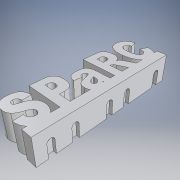
# Autodesk Inventor part: RGB Stand
Saved by Autodesk Inventor 2016 (Build 200138000, 138)
## iProperties
Created: 2015-11-06
Part Number: RGB Stand
Material: PPS Plastic
Document SubType Name: Modeling
Designer: Matthew
Density: 1.637 g/cm^3
Appearance: Smooth - White
Author: Matthew
## iProperties of the stored document RGB Stand_3DPrint.ipt
Created: 2015-11-06
Part Number: RGB Stand_3DPrint
Material: Generic
Document SubType Name: Modeling
Designer: Matthew
Density: 1 g/cm^3
Appearance: Default
Author: Matthew
Autodesk Inventor part; units mm, degrees
ref_plane "YZ Plane" through (0, 0, 0) normal (1, 0, 0) x (0, 1, 0)
ref_plane "XZ Plane" through (0, 0, 0) normal (0, 1, 0) x (-1, 0, 0)
ref_plane "XY Plane" through (0, 0, 0) normal (0, 0, 1) x (1, 0, 0)
sketch "Sketch1" plane through (0, 0, 0) normal (0, 1, 0) x (-1, 0, 0)
  line L0 (0, 0) -> (0, -279.4)
  line L1 (-0.0603, 0.0541) -> (-0.0603, -814.8468) construction
  line L2 (-0.0603, -814.8468) -> (-6674.4868, -814.8468) construction
  line L3 (-6674.4868, -814.8468) -> (-6674.4868, 0.0541) construction
  line L4 (-6674.4868, 0.0541) -> (-0.0603, 0.0541) construction
  line L5 (-49.463, -2.5788) -> (-48.1465, -18.4459)
  spline S0 degree 2 poles (-48.1465, -18.4459) (-53.3432, -18.9309) (-56.0454, -20.5246) knots 0 0 0 1 1 1
  spline S1 degree 2 poles (-56.0454, -20.5246) (-60.4106, -23.1575) (-60.4106, -27.9384) knots 0 0 0 1 1 1
  spline S2 degree 2 poles (-60.4106, -27.9384) (-60.4106, -31.4721) (-55.9068, -35.3523) (-52.9967, -35.3523) knots 0 0 0 1 2 2 2
  spline S3 degree 2 poles (-52.9967, -35.3523) (-50.2252, -35.3523) (-48.0079, -33.4815) knots 0 0 0 1 1 1
  spline S4 degree 2 poles (-48.0079, -33.4815) (-45.7907, -31.68) (-43.7813, -24.959) knots 0 0 0 1 1 1
  spline S5 degree 2 poles (-43.7813, -24.959) (-40.5248, -14.0114) (-35.051, -9.2998) knots 0 0 0 1 1 1
  spline S6 degree 2 poles (-35.051, -9.2998) (-29.5772, -4.5882) (-21.124, -4.5882) knots 0 0 0 1 1 1
  spline S7 degree 2 poles (-21.124, -4.5882) (-15.5809, -4.5882) (-5.742, -9.4384) (-0.0603, -19.1388) (-0.0603, -27.592) knots 0 0 0 1 2 3 3 3
  spline S8 degree 2 poles (-0.0603, -27.592) (-0.0603, -37.916) (-10.315, -48.7942) (-21.5398, -49.8336) knots 0 0 0 1 2 2 2
  line L6 (-21.5398, -49.8336) -> (-22.7869, -34.1051)
  spline S9 degree 2 poles (-22.7869, -34.1051) (-17.9368, -33.4815) (-13.5023, -29.4628) (-13.5023, -25.9291) knots 0 0 0 1 2 2 2
  spline S10 degree 2 poles (-13.5023, -25.9291) (-13.5023, -23.0189) (-16.7588, -20.0395) (-19.1839, -20.0395) knots 0 0 0 1 2 2 2
  spline S11 degree 2 poles (-19.1839, -20.0395) (-20.8469, -20.0395) (-22.2326, -21.2174) knots 0 0 0 1 1 1
  spline S12 degree 2 poles (-22.2326, -21.2174) (-23.6877, -22.3953) (-24.8656, -26.8298) knots 0 0 0 1 1 1
  spline S13 degree 2 poles (-24.8656, -26.8298) (-28.0529, -37.7774) (-34.4967, -47.2699) (-43.9892, -51.5658) (-49.8787, -51.5658) knots 0 0 0 1 2 3 3 3
  spline S14 degree 2 poles (-49.8787, -51.5658) (-56.8076, -51.5658) (-68.5173, -45.8148) (-74.5454, -35.4909) (-74.5454, -27.6613) knots 0 0 0 1 2 3 3 3
  spline S15 degree 2 poles (-74.5454, -27.6613) (-74.5454, -13.8729) (-60.4106, -3.2717) (-49.463, -2.5788) knots 0 0 0 1 2 2 2
  line L7 (-1.3075, -59.8804) -> (-1.3075, -87.5958)
  spline S16 degree 2 poles (-1.3075, -87.5958) (-1.3075, -96.6726) (-12.8094, -105.6801) (-23.4105, -105.6801) knots 0 0 0 1 2 2 2
  spline S17 degree 2 poles (-23.4105, -105.6801) (-34.3581, -105.6801) (-46.6222, -95.8411) (-46.6222, -85.7943) knots 0 0 0 1 2 2 2
  line L8 (-46.6222, -85.7943) -> (-46.6222, -76.6482)
  line L9 (-46.6222, -76.6482) -> (-73.2982, -76.6482)
  line L10 (-73.2982, -76.6482) -> (-73.2982, -59.8804)
  line L11 (-73.2982, -59.8804) -> (-1.3075, -59.8804)
  line L12 (-32.0023, -76.6482) -> (-32.0023, -80.7362)
  spline S18 degree 2 poles (-32.0023, -80.7362) (-32.0023, -85.5864) (-27.4986, -89.4666) (-24.0341, -89.4666) knots 0 0 0 1 2 2 2
  spline S19 degree 2 poles (-24.0341, -89.4666) (-20.639, -89.4666) (-15.9274, -86.0714) (-15.9274, -81.4291) knots 0 0 0 1 2 2 2
  line L13 (-15.9274, -81.4291) -> (-15.9274, -76.6482)
  line L14 (-15.9274, -76.6482) -> (-32.0023, -76.6482)
  line L15 (-38.0997, -127.0902) -> (-36.0903, -112.7475)
  spline S20 degree 2 poles (-36.0903, -112.7475) (-31.0323, -113.579) (-25.2813, -116.6276) (-23.1334, -119.4685) knots 0 0 0 1 2 2 2
  spline S21 degree 2 poles (-23.1334, -119.4685) (-21.609, -121.5471) (-19.9461, -128.7531) (-19.9461, -132.9797) knots 0 0 0 1 2 2 2
  spline S22 degree 2 poles (-19.9461, -132.9797) (-19.9461, -139.7007) (-21.9555, -147.8767) (-25.1428, -150.579) knots 0 0 0 1 2 2 2
  spline S23 degree 2 poles (-25.1428, -150.579) (-27.36, -152.5191) (-35.4667, -154.7363) (-39.139, -154.7363) knots 0 0 0 1 2 2 2
  line L16 (-39.139, -154.7363) -> (-62.2121, -154.7363)
  spline S24 degree 2 poles (-62.2121, -154.7363) (-65.8844, -154.7363) (-70.0417, -155.4292) (-73.2982, -156.6071) knots 0 0 0 1 2 2 2
  line L17 (-73.2982, -156.6071) -> (-73.2982, -142.6108)
  spline S25 degree 2 poles (-73.2982, -142.6108) (-71.2889, -141.7101) (-69.2102, -141.225) (-66.9237, -140.9479) knots 0 0 0 1 2 2 2
  spline S26 degree 2 poles (-66.9237, -140.9479) (-70.6653, -138.0378) (-72.3282, -135.1277) knots 0 0 0 1 1 1
  spline S27 degree 2 poles (-72.3282, -135.1277) (-74.4761, -131.1089) (-74.4761, -125.843) knots 0 0 0 1 1 1
  spline S28 degree 2 poles (-74.4761, -125.843) (-74.4761, -118.8449) (-65.8151, -111.5696) (-59.5098, -111.5696) knots 0 0 0 1 2 2 2
  spline S29 degree 2 poles (-59.5098, -111.5696) (-53.551, -111.5696) (-49.7402, -114.2025) knots 0 0 0 1 1 1
  spline S30 degree 2 poles (-49.7402, -114.2025) (-45.9293, -116.8355) (-44.0585, -123.8336) knots 0 0 0 1 1 1
  spline S31 degree 2 poles (-44.0585, -123.8336) (-41.772, -132.2868) (-39.9705, -137.3449) (-38.5154, -140.1164) knots 0 0 0 1 2 2 2
  spline S32 degree 2 poles (-38.5154, -140.1164) (-34.8431, -140.1164) (-31.8637, -137.8299) (-31.8637, -134.9198) knots 0 0 0 1 2 2 2
  spline S33 degree 2 poles (-31.8637, -134.9198) (-31.8637, -131.2475) (-33.4574, -129.446) knots 0 0 0 1 1 1
  spline S34 degree 2 poles (-33.4574, -129.446) (-34.7046, -127.991) (-38.0997, -127.0902) knots 0 0 0 1 1 1
  spline S35 degree 2 poles (-48.5623, -140.1164) (-50.0173, -136.9985) (-51.1952, -133.6726) knots 0 0 0 1 1 1
  spline S36 degree 2 poles (-51.1952, -133.6726) (-52.7888, -129.0996) (-54.3825, -127.8524) knots 0 0 0 1 1 1
  spline S37 degree 2 poles (-54.3825, -127.8524) (-55.9761, -126.6052) (-58.0548, -126.6052) knots 0 0 0 1 1 1
  spline S38 degree 2 poles (-58.0548, -126.6052) (-60.4106, -126.6052) (-63.39, -129.0996) (-63.39, -131.4554) knots 0 0 0 1 2 2 2
  spline S39 degree 2 poles (-63.39, -131.4554) (-63.39, -134.019) (-60.1334, -138.3149) (-55.4911, -140.1164) (-51.7495, -140.1164) knots 0 0 0 1 2 3 3 3
  line L18 (-51.7495, -140.1164) -> (-48.5623, -140.1164)
  line L19 (-73.2982, -164.9217) -> (-1.3075, -164.9217)
  line L20 (-1.3075, -164.9217) -> (-1.3075, -192.7064)
  spline S40 degree 2 poles (-1.3075, -192.7064) (-1.3075, -200.3974) (-4.8412, -208.5734) (-14.403, -213.5622) (-21.2626, -213.5622) knots 0 0 0 1 2 3 3 3
  spline S41 degree 2 poles (-21.2626, -213.5622) (-27.2907, -213.5622) (-35.9518, -209.7513) (-38.654, -206.4255) knots 0 0 0 1 2 2 2
  spline S42 degree 2 poles (-38.654, -206.4255) (-40.3862, -204.2775) (-41.4948, -200.536) knots 0 0 0 1 1 1
  spline S43 degree 2 poles (-41.4948, -200.536) (-42.8113, -203.5154) (-44.1278, -204.9011) knots 0 0 0 1 1 1
  spline S44 degree 2 poles (-44.1278, -204.9011) (-45.0285, -205.8019) (-50.8488, -209.3356) (-52.3731, -209.8899) knots 0 0 0 1 2 2 2
  line L21 (-52.3731, -209.8899) -> (-73.2982, -217.9274)
  line L22 (-73.2982, -217.9274) -> (-73.2982, -199.0809)
  line L23 (-73.2982, -199.0809) -> (-51.2645, -190.212)
  spline S45 degree 2 poles (-51.2645, -190.212) (-47.0379, -188.5491) (-45.7214, -187.2326) knots 0 0 0 1 1 1
  spline S46 degree 2 poles (-45.7214, -187.2326) (-44.0585, -185.4311) (-44.0585, -183.1446) knots 0 0 0 1 1 1
  line L24 (-44.0585, -183.1446) -> (-44.0585, -181.6895)
  line L25 (-44.0585, -181.6895) -> (-73.2982, -181.6895)
  line L26 (-73.2982, -181.6895) -> (-73.2982, -164.9217)
  line L27 (-30.478, -181.6895) -> (-30.478, -188.6876)
  spline S47 degree 2 poles (-30.478, -188.6876) (-30.478, -189.7963) (-29.5079, -193.0528) knots 0 0 0 1 1 1
  spline S48 degree 2 poles (-29.5079, -193.0528) (-29.0229, -194.7157) (-25.4199, -196.7944) (-23.0641, -196.7944) knots 0 0 0 1 2 2 2
  spline S49 degree 2 poles (-23.0641, -196.7944) (-19.5997, -196.7944) (-15.8581, -193.5378) (-15.8581, -188.9648) knots 0 0 0 1 2 2 2
  line L28 (-15.8581, -188.9648) -> (-15.8581, -181.6895)
  line L29 (-15.8581, -181.6895) -> (-30.478, -181.6895)
  line L30 (-43.8506, -259.2926) -> (-49.7402, -273.9124)
  spline S50 degree 2 poles (-49.7402, -273.9124) (-57.9162, -272.4574) (-68.9331, -266.0829) (-74.5454, -256.7289) (-74.5454, -249.5229) knots 0 0 0 1 2 3 3 3
  spline S51 degree 2 poles (-74.5454, -249.5229) (-74.5454, -240.7233) (-67.6859, -229.5678) (-50.5023, -221.4611) (-37.1297, -221.4611) knots 0 0 0 1 2 3 3 3
  spline S52 degree 2 poles (-37.1297, -221.4611) (-19.2532, -221.4611) (-0.0603, -235.7345) (-0.0603, -248.7607) knots 0 0 0 1 2 2 2
  spline S53 degree 2 poles (-0.0603, -248.7607) (-0.0603, -258.9461) (-11.0772, -270.5866) (-22.4405, -273.4274) knots 0 0 0 1 2 2 2
  line L31 (-22.4405, -273.4274) -> (-26.8057, -258.669)
  spline S54 degree 2 poles (-26.8057, -258.669) (-23.5491, -257.9068) (-22.0248, -257.0754) knots 0 0 0 1 1 1
  spline S55 degree 2 poles (-22.0248, -257.0754) (-19.4611, -255.6896) (-16.6896, -251.6016) (-16.6896, -249.1072) knots 0 0 0 1 2 2 2
  spline S56 degree 2 poles (-16.6896, -249.1072) (-16.6896, -243.4255) (-22.7869, -240.4461) knots 0 0 0 1 1 1
  spline S57 degree 2 poles (-22.7869, -240.4461) (-27.2907, -238.1596) (-36.9911, -238.1596) knots 0 0 0 1 1 1
  spline S58 degree 2 poles (-36.9911, -238.1596) (-48.978, -238.1596) (-57.8469, -243.6334) (-57.8469, -248.5529) knots 0 0 0 1 2 2 2
  spline S59 degree 2 poles (-57.8469, -248.5529) (-57.8469, -253.3338) (-50.7102, -258.184) (-43.8506, -259.2926) knots 0 0 0 1 2 2 2
  dimension "d0" = 279.4
  constraints: 2 end point, 1 vertical, 2 other
  measures "d0" distance of L0.start L0.end
extrude "Extrusion1" add sketch "Sketch1" along normal blind 50.8
sketch "Sketch5" plane through (0, 50.8, 0) normal (0, 1, 0) x (1, 0, 0)
  line L0 (48.1465, 18.4459) -> (49.463, 2.5788) projected
  line L1 (22.7869, 34.1051) -> (21.5398, 49.8336) projected
  line L2 (32.0023, 76.6482) -> (15.9274, 76.6482) projected
  line L3 (15.9274, 76.6482) -> (15.9274, 81.4291) projected
  line L4 (32.0023, 80.7362) -> (32.0023, 76.6482) projected
  line L5 (1.3075, 87.5958) -> (1.3075, 59.8804) projected
  line L6 (1.3075, 59.8804) -> (73.2982, 59.8804) projected
  line L7 (73.2982, 59.8804) -> (73.2982, 76.6482) projected
  line L8 (73.2982, 76.6482) -> (46.6222, 76.6482) projected
  line L9 (46.6222, 76.6482) -> (46.6222, 85.7943) projected
  line L10 (48.5623, 140.1164) -> (51.7495, 140.1164) projected
  line L11 (36.0903, 112.7475) -> (38.0997, 127.0902) projected
  line L12 (73.2982, 142.6108) -> (73.2982, 156.6071) projected
  line L13 (62.2121, 154.7363) -> (39.139, 154.7363) projected
  line L14 (30.478, 181.6895) -> (15.8581, 181.6895) projected
  line L15 (15.8581, 181.6895) -> (15.8581, 188.9648) projected
  line L16 (30.478, 188.6876) -> (30.478, 181.6895) projected
  line L17 (1.3075, 164.9217) -> (73.2982, 164.9217) projected
  line L18 (73.2982, 164.9217) -> (73.2982, 181.6895) projected
  line L19 (73.2982, 181.6895) -> (44.0585, 181.6895) projected
  line L20 (44.0585, 181.6895) -> (44.0585, 183.1446) projected
  line L21 (51.2645, 190.212) -> (73.2982, 199.0809) projected
  line L22 (73.2982, 199.0809) -> (73.2982, 217.9274) projected
  line L23 (73.2982, 217.9274) -> (52.3731, 209.8899) projected
  line L24 (1.3075, 192.7064) -> (1.3075, 164.9217) projected
  line L25 (49.7402, 273.9124) -> (43.8506, 259.2926) projected
  line L26 (26.8057, 258.669) -> (22.4405, 273.4274) projected
  line L27 (48.1465, 18.4459) -> (49.463, 2.5788) projected
  line L28 (49.463, 2.5788) -> (96.7361, 2.5788)
  line L29 (49.7402, 273.9124) -> (43.8506, 259.2926) projected
  line L30 (49.7402, 273.9124) -> (101.1654, 273.9124)
  line L31 (87.2454, 27.6613) -> (87.2454, 2.5788)
  line L32 (68.6857, 2.5788) -> (68.6857, 273.9124)
  line L33 (87.2454, 2.5788) -> (87.2454, 273.9124)
  point P0 (0, 0)
  constraints: 10 end point, 5 point on line, 2 horizontal, 2 perpendicular, 60 other
extrude "Extrusion3" add sketch "Sketch5" against normal blind 50.8
sketch "Sketch6" plane through (87.2454, 50.8, -2.5788) normal (1, 0, 0) x (0, 0, -1)
  line L0 (0, 0) -> (271.3336, 0) projected
  line L1 (0, 0) -> (0, -50.8) projected
  line L2 (271.3336, -50.8) -> (0, -50.8) projected
  line L3 (271.3336, 0) -> (271.3336, -50.8) projected
  line L4 (87.2454, -50.8) -> (87.2454, 0) projected
  line L5 (87.2454, 0) -> (87.2454, -50.8) projected
  line L6 (57.3016, -50.8) -> (57.3016, 0) projected
  line L7 (74.0694, 0) -> (74.0694, -50.8) projected
  line L8 (87.2454, -50.8) -> (87.2454, 0) projected
  line L9 (87.2454, 0) -> (87.2454, -50.8) projected
  line L10 (162.3429, -50.8) -> (162.3429, 0) projected
  line L11 (179.1107, 0) -> (179.1107, -50.8) projected
  line L12 (87.2454, -50.8) -> (87.2454, 0) projected
  line L13 (87.2454, 0) -> (87.2454, -50.8) projected
  line L14 (111.6237, -50.8) -> (111.6237, 0) projected
  line L15 (152.1575, -50.8) -> (152.1575, 0) projected
  line L16 (87.2454, -25.4) -> (87.2454, -25.4)
  arc A0 (28.5346, -25.4) -> (22.1846, -25.4) centre (25.3596, -25.4) ccw
  circle A1 centre (65.6855, -25.4) radius 3.175
  circle A2 centre (131.6232, -25.3318) radius 3.175
  circle A3 centre (170.7268, -25.4) radius 3.175
  circle A4 centre (246.0842, -25.4) radius 3.175
  arc A5 (31.7096, -25.4) -> (19.0096, -25.4) centre (25.3596, -25.4) ccw
  arc A6 (72.0355, -25.4) -> (59.3355, -25.4) centre (65.6855, -25.4) ccw
  arc A7 (137.9728, -25.2651) -> (125.2735, -25.3986) centre (131.6232, -25.3318) ccw
  arc A8 (177.0768, -25.4) -> (164.3768, -25.4) centre (170.7268, -25.4) ccw
  arc A9 (252.4342, -25.4) -> (239.7342, -25.4) centre (246.0842, -25.4) ccw
  line L17 (19.0096, -25.4) -> (19.0096, -50.8)
  line L18 (271.3336, -50.8) -> (0, -50.8) projected
  line L19 (31.7096, -25.4) -> (31.7096, -50.8)
  line L20 (59.3355, -25.4) -> (59.3355, -50.8)
  line L21 (72.0355, -25.4) -> (72.0355, -50.8)
  line L22 (125.2735, -50.8) -> (125.2735, 0) projected
  line L23 (125.2735, -25.4) -> (125.2735, -50.8)
  line L24 (138.3691, -50.8) -> (138.3691, 0) projected
  line L25 (137.9728, -25.2651) -> (138.3691, -50.8)
  line L26 (164.3768, -25.4) -> (164.3768, -50.8)
  line L27 (177.0768, -25.4) -> (177.0768, -50.8)
  line L28 (239.7342, -25.4) -> (239.7342, -50.8)
  line L29 (252.4342, -25.4) -> (252.4342, -50.8)
  arc A10 (22.1846, -25.4) -> (28.5346, -25.4) centre (25.3596, -25.4) ccw
  line L30 (125.2735, -25.3986) -> (125.2735, -50.8)
  point P0 (-2.5788, -50.8)
  point P1 (7.0095, -50.8)
  point P2 (7.0095, 0)
  point P3 (41.8171, 0)
  point P4 (41.8171, -50.8)
  point P5 (111.542, -50.8)
  point P6 (111.542, 0)
  point P7 (152.6419, 0)
  point P8 (152.6419, -50.8)
  point P9 (229.453, -50.8)
  point P10 (229.453, 0)
  point P11 (262.7155, 0)
  point P12 (262.7155, -50.8)
  dimension "d10" = 6.35
  dimension "d11" = 6.35
  dimension "d12" = 6.35
  dimension "d13" = 6.35
  dimension "d14" = 6.35
  dimension "d15" = 12.7
  dimension "d16" = 12.7
  dimension "d17" = 12.7
  dimension "d18" = 12.7
  dimension "d19" = 12.7
  constraints: 24 end point, 14 point on circle, 11 centre point, 6 tangent, 5 coincident, 5 parallel, 4 vertical, 3 point on line, 2 vertical alignment, 1 collinear, 1 midpoint, 15 other
  measures "d10" diameter of A0
  measures "d11" diameter of A1
  measures "d12" diameter of A2
  measures "d13" diameter of A3
  measures "d14" diameter of A4
  measures "d15" diameter of A5
  measures "d16" diameter of A6
  measures "d17" diameter of A7
  measures "d18" diameter of A8
  measures "d19" diameter of A9
extrude "Extrusion4" cut sketch "Sketch6" against normal blind 6.35 contours L17 A5 L19 L2 | L20 A6 L21 L2 | A7 L25 L2 L22 | L26 A8 L27 L2 | L28 A9 L29 L2
sketch "Sketch7" plane through (87.2454, 25.4, -27.9384) normal (1, 0, 0) x (0, 0, -1)
  circle A0 centre (0, 0) radius 3.175 projected
  circle A1 centre (40.3259, 0) radius 3.175 projected
  circle A2 centre (106.2636, 0.0682) radius 3.175 projected
  circle A3 centre (145.3672, 0) radius 3.175 projected
  circle A4 centre (220.7247, 0) radius 3.175 projected
  point P0 (-27.9384, -25.4)
extrude "Extrusion5" cut sketch "Sketch7" against normal blind 12.7
body "Solid1"
